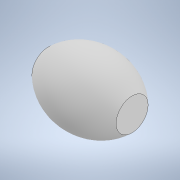
# Autodesk Inventor part: N4
Saved by Autodesk Inventor 2022 (Build 260153000, 153)
## iProperties
Created: 2023-03-30
Part Number: N4
Material: Типовые
Document SubType Name: Modeling
Designer: Hp
Density: 1 g/cm^3
Appearance: По умолчанию
Author: Hp
Autodesk Inventor part; units mm, degrees
ref_plane "YZ Plane" through (0, 0, 0) normal (1, 0, 0) x (0, 1, 0)
ref_plane "XZ Plane" through (0, 0, 0) normal (0, 1, 0) x (-1, 0, 0)
ref_plane "XY Plane" through (0, 0, 0) normal (0, 0, 1) x (1, 0, 0)
sketch "Эскиз1" plane through (0, 0, 0) normal (0, 0, 1) x (1, 0, 0)
  line L0 (0, 0) -> (40, 0)
  arc A0 (40, 7.5959) -> (0, 7.5959) centre (20, -12) ccw
  line L1 (0, 0) -> (0, 7.5959)
  line L2 (40, 0) -> (40, 7.5959)
  dimension "d0" = 40
  dimension "d5" = 28
  constraints: 6 end point, 2 point on circle, 1 centre point, 1 horizontal, 1 parallel, 1 vertical
  measures "d0" distance of L0.start L0.end
  measures "d5" radius of A0
revolve "Вращение1" add sketch "Эскиз1" angle 360 about axis through (0, 0, 0) along (1, 0, 0)
